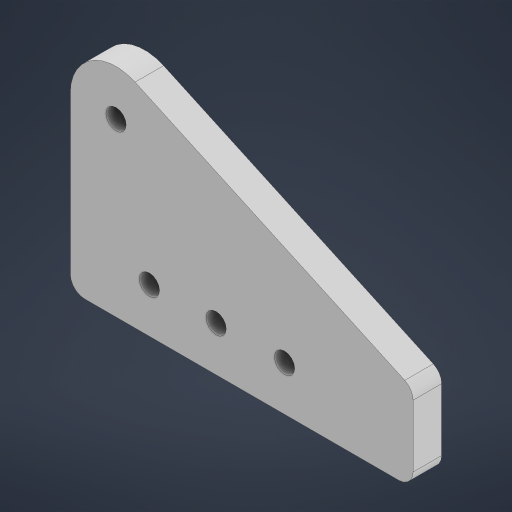
# Autodesk Inventor part: Slide_Climb_Conforce_Spring_Mount
Saved by Autodesk Inventor 2023 (Build 270158000, 158)
## iProperties
Created: 2024-02-27
Part Number: Slide_Climb_Conforce_Spring_Mount
Material: Generic
Document SubType Name: Modeling
Designer: kelle
Density: 1 g/cm^3
Appearance: Default
Mass: 25.8397 g
Surface Area: 106.569 cm^2
Volume: 25.8397 cm^3
Author: kelle
Autodesk Inventor part; units mm, degrees
ref_plane "YZ Plane" through (0, 0, 0) normal (1, 0, 0) x (0, 1, 0)
ref_plane "XZ Plane" through (0, 0, 0) normal (0, 1, 0) x (-1, 0, 0)
ref_plane "XY Plane" through (0, 0, 0) normal (0, 0, 1) x (1, 0, 0)
sketch "Sketch1" plane through (0, 0, 0) normal (0, 0, 1) x (1, 0, 0)
  line L0 (38.1, -19.05) -> (-38.1, -19.05)
  line L1 (-38.1, -19.05) -> (-38.1, 19.05)
  line L2 (-38.1, 19.05) -> (38.1, 19.05)
  line L3 (38.1, 19.05) -> (38.1, -19.05)
  line L4 (38.1, -19.05) -> (-38.1, 19.05) construction
  line L5 (-38.1, -19.05) -> (38.1, 19.05) construction
  line L6 (-38.1, -19.05) -> (38.1, -19.05)
  line L7 (38.1, -19.05) -> (38.1, 0.8382)
  line L8 (38.1, 0.8382) -> (-38.1, 0.8382) construction
  line L9 (-38.1, 0.8382) -> (-38.1, -19.05)
  line L10 (-38.1, -9.1059) -> (38.1, -9.1059) construction
  circle A0 centre (-20.5232, -9.1059) radius 2.25
  circle A1 centre (-5.6896, -9.1059) radius 2.25
  circle A2 centre (9.525, -9.1059) radius 2.25
  circle A3 centre (-27.94, 19.05) radius 6.35 construction
  circle A4 centre (-27.94, 19.05) radius 2.25
  circle A5 centre (-27.94, 19.05) radius 10.16
  line L11 (38.1, 0) -> (-23.712, 28.2885)
  point P0 (0, 0)
  point P1 (-38.1, 19.05)
  point P2 (-17.78, 19.05)
  point P3 (-3.5254, 19.05)
  dimension "d0" = 76.2
  dimension "d1" = 38.1
  dimension "d2" = 19.8882
  dimension "d3" = 4.5
  dimension "d4" = 17.5768
  dimension "d5" = 4.5
  dimension "d6" = 14.8336
  dimension "d7" = 4.5
  dimension "d8" = 15.2146
  dimension "d9" = 12.7
  dimension "d10" = 0
  dimension "d11" = 10.16
  dimension "d12" = 4.5
  constraints: 24 end point, 5 centre point, 5 point on line, 4 midpoint, 4 parallel, 2 coincident, 2 horizontal, 2 perpendicular, 1 vertical, 4 other
  measures "d0" distance of L1.end L2.end
  measures "d1" distance of L0.end L1.end
  measures "d2" distance of L7.end L6.end
  measures "d3" diameter of A0
  measures "d4" distance from line of L1 A0.centre
  measures "d5" diameter of A1
  measures "d6" distance of A0.centre A1.centre
  measures "d7" diameter of A2
  measures "d8" distance of A1.centre A2.centre
  measures "d9" diameter of A3
  measures "d10" distance from line of L2 A3.centre
  measures "d11" distance from line of L1 A3.centre
  measures "d12" diameter of A4
extrude "Extrusion1" add sketch "Sketch1" along normal blind 6.35 contours L0 L1 A5 L2 L11 L3 | L11 L2 L3 | L2 A5 L11 | A5 L2 A4 | L2 A4 A5
extrude "Extrusion2" cut sketch "Sketch1" along normal blind 6.35 contours L11 L2 L3
fillet "Fillet1" radius 3.175 2 edges at (38.1, -19.05, 3.175) (-38.1, -19.05, 3.175)
body "Solid1"
